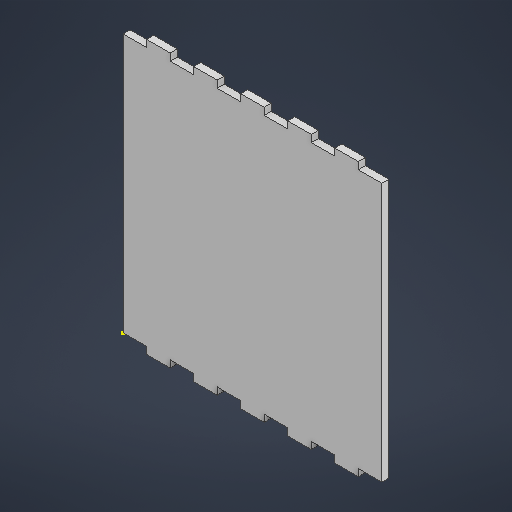
# Autodesk Inventor part: Techopantalla
Saved by Autodesk Inventor 2026 (Build 300175000, 175)
## iProperties
Created: 2026-04-21
Part Number: Techopantalla
Material: Generic
Document SubType Name: Modeling
Designer: juana
Density: 1 g/cm^3
Appearance: Default
Author: juana
Autodesk Inventor part; units mm, degrees
ref_plane "YZ Plane" through (0, 0, 0) normal (1, 0, 0) x (0, 1, 0)
ref_plane "XZ Plane" through (0, 0, 0) normal (0, 1, 0) x (-1, 0, 0)
ref_plane "XY Plane" through (0, 0, 0) normal (0, 0, 1) x (1, 0, 0)
sketch "Sketch1" plane through (0, 0, 0) normal (0, 0, 1) x (1, 0, 0)
  line L0 (0, 0) -> (110, 0)
  line L1 (110, 0) -> (110, 110)
  line L2 (110, 110) -> (0, 110)
  line L3 (0, 110) -> (0, 0)
  dimension "d0" = 110
  dimension "d1" = 110
  constraints: 8 end point, 2 parallel, 1 horizontal, 1 perpendicular
  measures "d0" distance of L0.start L0.end
  measures "d1" distance of L2.end L0.start
extrude "Extrusion1" add sketch "Sketch1" along normal blind 3
sketch "Sketch2" plane through (0, 0, 3) normal (0, 0, 1) x (1, 0, 0)
  line L0 (110, 110) -> (0, 110) projected
  line L1 (10, 110) -> (20, 110)
  line L2 (20, 110) -> (20, 113)
  line L3 (20, 113) -> (10, 113)
  line L4 (10, 113) -> (10, 110)
  line L5 (30, 110) -> (40, 110)
  line L6 (40, 110) -> (40, 113)
  line L7 (40, 113) -> (30, 113)
  line L8 (30, 113) -> (30, 110)
  line L9 (50, 110) -> (60, 110)
  line L10 (60, 110) -> (60, 113)
  line L11 (60, 113) -> (50, 113)
  line L12 (50, 113) -> (50, 110)
  line L13 (70, 110) -> (80, 110)
  line L14 (80, 110) -> (80, 113)
  line L15 (80, 113) -> (70, 113)
  line L16 (70, 113) -> (70, 110)
  line L17 (90, 110) -> (100, 110)
  line L18 (100, 110) -> (100, 113)
  line L19 (100, 113) -> (90, 113)
  line L20 (90, 113) -> (90, 110)
  line L21 (0, 110) -> (0, 0) projected
  line L22 (10, -3) -> (20, -3)
  line L23 (20, -3) -> (20, 0)
  line L24 (20, 0) -> (10, 0)
  line L25 (10, 0) -> (10, -3)
  line L26 (30, -3) -> (40, -3)
  line L27 (40, -3) -> (40, 0)
  line L28 (40, 0) -> (30, 0)
  line L29 (30, 0) -> (30, -3)
  line L30 (50, -3) -> (60, -3)
  line L31 (60, -3) -> (60, 0)
  line L32 (60, 0) -> (50, 0)
  line L33 (50, 0) -> (50, -3)
  line L34 (70, -3) -> (80, -3)
  line L35 (80, -3) -> (80, 0)
  line L36 (80, 0) -> (70, 0)
  line L37 (70, 0) -> (70, -3)
  line L38 (90, -3) -> (100, -3)
  line L39 (100, -3) -> (100, 0)
  line L40 (100, 0) -> (90, 0)
  line L41 (90, 0) -> (90, -3)
  dimension "d4" = 10
  dimension "d5" = 3
  dimension "d6" = 10
  dimension "d9" = 20
  dimension "d12" = 113
  constraints: 80 end point, 2 horizontal, 2 parallel, 1 perpendicular, 1 point on line, 1 vertical, 72 other
  measures "d4" distance of L2.end L3.end
  measures "d5" distance of L1.end L2.end
  measures "d6" distance from line of L0.end L4
  measures "d9" distance of L1.start L5.start
  measures "d12" distance of L1.start L22.start
extrude "Extrusion2" add sketch "Sketch2" against normal blind 3
sketch "Sketch3" plane through (0, 0, 3) normal (0, 0, 1) x (1, 0, 0)
  point P0 (0, 0)
body "Solid1"
